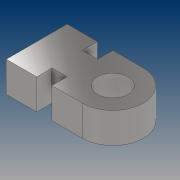
# Autodesk Inventor part: 32
Saved by Autodesk Inventor 2020.2 (Build 242310000, 310)
## iProperties
Created: 2020-09-17
Part Number: 32
Material: 鋼、碳鋼
Document SubType Name: Modeling
Designer: user
Density: 7.85 g/cm^3
Appearance: 半拋光
Mass: 331.923 g
Surface Area: 103.416 cm^2
Volume: 42.2832 cm^3
Author: user
Autodesk Inventor part; units mm, degrees
ref_plane "YZ Plane" through (0, 0, 0) normal (1, 0, 0) x (0, 1, 0)
ref_plane "XZ Plane" through (0, 0, 0) normal (0, 1, 0) x (-1, 0, 0)
ref_plane "XY Plane" through (0, 0, 0) normal (0, 0, 1) x (1, 0, 0)
sketch "草圖1" plane through (0, 0, 0) normal (0, 1, 0) x (-1, 0, 0)
  circle A0 centre (0, 0) radius 20
  line L0 (0, -20) -> (50, -20)
  line L1 (50, -20) -> (50, 20)
  line L2 (50, 20) -> (0, 20)
  line L3 (0, 20) -> (0, -20)
  point P0 (0, 20)
  dimension "d0" = 40
  dimension "d1" = 50
  constraints: 8 end point, 3 horizontal, 2 parallel, 1 coincident, 1 perpendicular, 3 other
  measures "d1" distance of L0.start L0.end
extrude "擠出1" add sketch "草圖1" along normal blind 20
sketch "草圖2" plane through (0, 20, 0) normal (0, 1, 0) x (1, 0, 0)
  line L0 (-50, -20) -> (-50, 20) projected
  line L1 (-50, 20) -> (0, 20) projected
  arc A0 (0, -20) -> (0, 20) centre (0, 0) ccw projected
  line L2 (0, -20) -> (-50, -20) projected
  line L3 (-30, -10) -> (-20, -10)
  line L4 (-20, -10) -> (-20, -20)
  line L5 (-20, -20) -> (-30, -20)
  line L6 (-30, -20) -> (-30, -10)
  line L7 (-50, -20) -> (0, -20) projected
  dimension "d4" = 10
  dimension "d5" = 10
  dimension "d6" = 20
  constraints: 8 end point, 2 parallel, 1 collinear, 1 horizontal, 1 perpendicular
  measures "d4" distance of L3.start L3.end
  measures "d5" distance of L5.end L3.start
  measures "d6" distance between parallel lines of L6 L0
extrude "擠出2" cut sketch "草圖2" against normal through all contours L6 L3 L4 L2
mirror "鏡射1" about plane through (0, 0, 0) normal (0, 0, 1) of "擠出2"
sketch "草圖3" plane through (0, 20, 0) normal (0, 1, 0) x (1, 0, 0)
  arc A0 (0, -20) -> (0, 20) centre (0, 0) ccw projected
  constraints: 1 coincident
hole "孔1" at (0, 20, 0) direction (0, -1, 0) diameter 20 end through all
